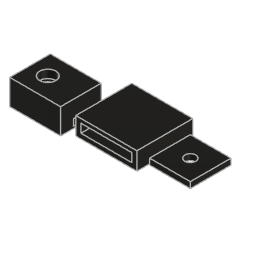
fit-coupons (Autodesk Fusion 360 design; units mm, degrees)
description: Fit sample only; a 25 mm screw will protrude through this shorter coupon
description: Insert measured acrylic from the open end; check emitting centre against edge
description: Test the actual printed reset stem in this 4.3 mm bore
Autodesk Fusion 360 part; units mm, degrees
sketch "Fastener test block profile" plane through (0, 0, 0) normal (0, 0, 1) x (1, 0, 0) in component "90 M3 head and nut fit sample"
  line L0 (0, 0) -> (20, 0)
  line L1 (20, 0) -> (20, 16)
  line L2 (20, 16) -> (0, 16)
  line L3 (0, 16) -> (0, 0)
  dimension "d44" = 20
  dimension "d45" = 16
  measures "d44" horizontal distance of L0.start L0.end
  measures "d45" vertical distance of L0.end L1.end
extrude "Fastener test block" add sketch "Fastener test block profile" against normal blind 10 makes body 1 in component "90 M3 head and nut fit sample"
sketch "M3 clearance profile" plane through (0, 0, 0) normal (0, 0, 1) x (1, 0, 0) in component "90 M3 head and nut fit sample"
  circle A0 centre (7, 8) radius 1.7
  dimension "d48" = 3.4
  measures "d48" diameter of A0
extrude "M3 clearance" cut sketch "M3 clearance profile" against normal blind 10 bodies 1 in component "90 M3 head and nut fit sample"
sketch "M3 head recess profile" plane through (0, 0, 0) normal (0, 0, 1) x (1, 0, 0) in component "90 M3 head and nut fit sample"
  circle A0 centre (7, 8) radius 3.2
  dimension "d51" = 6.4
  measures "d51" diameter of A0
extrude "M3 head recess" cut sketch "M3 head recess profile" against normal blind 3.2 bodies 1 in component "90 M3 head and nut fit sample"
ref_plane "WorkPlane1" through (0, 0, -6.6) normal (0, 0, 1) x (1, 0, 0) in component "90 M3 head and nut fit sample"
sketch "Nut sample hex" plane through (0, 0, -6.6) normal (0, 0, 1) x (1, 0, 0) in component "90 M3 head and nut fit sample"
  line L0 (10.3486, 8) -> (8.6743, 10.9)
  line L1 (8.6743, 10.9) -> (5.3257, 10.9)
  line L2 (5.3257, 10.9) -> (3.6514, 8)
  line L3 (3.6514, 8) -> (5.3257, 5.1)
  line L4 (5.3257, 5.1) -> (8.6743, 5.1)
  line L5 (8.6743, 5.1) -> (10.3486, 8)
extrude "Nut pocket" cut sketch "Nut sample hex" against normal blind 2.6 bodies 1 in component "90 M3 head and nut fit sample"
ref_plane "WorkPlane2" through (0, 0, -6.6) normal (0, 0, 1) x (1, 0, 0) in component "90 M3 head and nut fit sample"
sketch "Side nut loading slot profile" plane through (0, 0, -6.6) normal (0, 0, 1) x (1, 0, 0) in component "90 M3 head and nut fit sample"
  line L0 (7, 5.1) -> (20, 5.1)
  line L1 (20, 5.1) -> (20, 10.9)
  line L2 (20, 10.9) -> (7, 10.9)
  line L3 (7, 10.9) -> (7, 5.1)
  dimension "d60" = 13
  dimension "d61" = 5.8
  measures "d60" horizontal distance of L0.start L0.end
  measures "d61" vertical distance of L0.end L1.end
extrude "Side nut loading slot" cut sketch "Side nut loading slot profile" against normal blind 2.6 bodies 1 in component "90 M3 head and nut fit sample"
sketch "Optical test block profile" plane through (0, 0, 0) normal (0, 0, 1) x (1, 0, 0) in component "91 LED and acrylic fit sample"
  line L0 (26, 0) -> (50, 0)
  line L1 (50, 0) -> (50, 22)
  line L2 (50, 22) -> (26, 22)
  line L3 (26, 22) -> (26, 0)
  dimension "d64" = 24
  dimension "d65" = 22
  measures "d64" horizontal distance of L0.start L0.end
  measures "d65" vertical distance of L0.end L1.end
extrude "Optical test block" add sketch "Optical test block profile" against normal blind 7 separate body makes body 2 in component "91 LED and acrylic fit sample"
ref_plane "WorkPlane1" through (0, 0, -1.6) normal (0, 0, 1) x (1, 0, 0) in component "91 LED and acrylic fit sample"
sketch "Acrylic slip slot profile" plane through (0, 0, -1.6) normal (0, 0, 1) x (1, 0, 0) in component "91 LED and acrylic fit sample"
  line L0 (28, -0.1) -> (48, -0.1)
  line L1 (48, -0.1) -> (48, 12.2)
  line L2 (48, 12.2) -> (28, 12.2)
  line L3 (28, 12.2) -> (28, -0.1)
  dimension "d70" = 20
  dimension "d71" = 12.3
  measures "d70" horizontal distance of L0.start L0.end
  measures "d71" vertical distance of L0.end L1.end
extrude "Acrylic slip slot" cut sketch "Acrylic slip slot profile" against normal blind 3.425 bodies 2 in component "91 LED and acrylic fit sample"
ref_plane "WorkPlane2" through (0, 0, -2.1875) normal (0, 0, 1) x (1, 0, 0) in component "91 LED and acrylic fit sample"
sketch "LED open rear pocket profile" plane through (0, 0, -2.1875) normal (0, 0, 1) x (1, 0, 0) in component "91 LED and acrylic fit sample"
  line L0 (33.8, 12.2) -> (42.2, 12.2)
  line L1 (42.2, 12.2) -> (42.2, 20.6)
  line L2 (42.2, 20.6) -> (33.8, 20.6)
  line L3 (33.8, 20.6) -> (33.8, 12.2)
  dimension "d76" = 8.4
  dimension "d77" = 8.4
  measures "d76" horizontal distance of L0.start L0.end
  measures "d77" vertical distance of L0.end L1.end
extrude "LED open rear pocket" cut sketch "LED open rear pocket profile" against normal blind 5 bodies 2 in component "91 LED and acrylic fit sample"
ref_plane "WorkPlane3" through (0, 0, -1.6) normal (0, 0, 1) x (1, 0, 0) in component "91 LED and acrylic fit sample"
sketch "Optical entry aperture profile" plane through (0, 0, -1.6) normal (0, 0, 1) x (1, 0, 0) in component "91 LED and acrylic fit sample"
  line L0 (33.8, 11.9) -> (42.2, 11.9)
  line L1 (42.2, 11.9) -> (42.2, 12.3)
  line L2 (42.2, 12.3) -> (33.8, 12.3)
  line L3 (33.8, 12.3) -> (33.8, 11.9)
  dimension "d82" = 8.4
  dimension "d83" = 0.4
  measures "d82" horizontal distance of L0.start L0.end
  measures "d83" vertical distance of L0.end L1.end
extrude "Optical entry aperture" cut sketch "Optical entry aperture profile" against normal blind 3.425 bodies 2 in component "91 LED and acrylic fit sample"
sketch "Plunger guide block profile" plane through (0, 0, 0) normal (0, 0, 1) x (1, 0, 0) in component "92 Reset guide fit sample"
  line L0 (55, 0) -> (71, 0)
  line L1 (71, 0) -> (71, 16)
  line L2 (71, 16) -> (55, 16)
  line L3 (55, 16) -> (55, 0)
  dimension "d86" = 16
  dimension "d87" = 16
  measures "d86" horizontal distance of L0.start L0.end
  measures "d87" vertical distance of L0.end L1.end
extrude "Plunger guide block" add sketch "Plunger guide block profile" against normal blind 2.4 separate body makes body 3 in component "92 Reset guide fit sample"
sketch "Stem guide clearance profile" plane through (0, 0, 0) normal (0, 0, 1) x (1, 0, 0) in component "92 Reset guide fit sample"
  circle A0 centre (63, 8) radius 2.15
  dimension "d90" = 4.3
  measures "d90" diameter of A0
extrude "Stem guide clearance" cut sketch "Stem guide clearance profile" against normal blind 2.4 bodies 3 in component "92 Reset guide fit sample"
component "90 M3 head and nut fit sample" placed x (1, 0, 0) y (0, 1, 0) z (0, 0, 1) at (0, 0, 0)
component "91 LED and acrylic fit sample" placed x (1, 0, 0) y (0, 1, 0) z (0, 0, 1) at (0, 0, 0)
component "92 Reset guide fit sample" placed x (1, 0, 0) y (0, 1, 0) z (0, 0, 1) at (0, 0, 0)
equation "case_w = 120.0000000 mm" comment "Overall width"
equation "case_h = 60.0000000 mm" comment "Overall height"
equation "case_d = 30.0000000 mm" comment "Overall depth; excludes adhesive strips"
equation "wall = 2.4000000 mm" comment "PETG wall thickness"
equation "front_lip = 1.6000000 mm" comment "Front retaining lip"
equation "window_w = 100.0000000 mm" comment "Visible opening width"
equation "window_h = 34.0000000 mm" comment "Visible opening height"
equation "panel_w = 104.0000000 mm" comment "Keyed optical panel width"
equation "panel_h = 38.0000000 mm" comment "Keyed optical panel height"
equation "acrylic_t = 3.1750000 mm" comment "MEASURE: actual sheet thickness"
equation "air_gap = 0.5000000 mm" comment "Clearance from engraving to raised white letters"
equation "backing_base = 1.6000000 mm" comment "Black backing base thickness"
equation "letter_relief = 0.4000000 mm" comment "White final two 0.2 mm layers"
equation "tray_t = 1.6000000 mm" comment "Optical support and electronics tray base"
equation "fit = 0.2500000 mm" comment "Sliding fit allowance per side; verify with coupon"
equation "led_w = 8.0000000 mm" comment "MEASURE: individual LED PCB width"
equation "led_h = 8.0000000 mm" comment "MEASURE: individual LED PCB length"
equation "led_t = 2.0000000 mm" comment "MEASURE: LED assembly depth"
equation "led_face_gap = 0.2000000 mm" comment "Emitter to acrylic edge gap"
equation "led_optical_offset = 1.0000000 mm" comment "MEASURE: emitter centre from frontmost module surface"
equation "battery_w = 52.0000000 mm" comment "Supplied battery width"
equation "battery_h = 21.0000000 mm" comment "Supplied battery height"
equation "battery_t = 10.0000000 mm" comment "Supplied battery thickness"
equation "charger_w = 16.5000000 mm" comment "Listed board width; confirm physical board"
equation "charger_h = 25.0000000 mm" comment "Listed board length; confirm physical board"
equation "charger_pcb_t = 1.0000000 mm" comment "MEASURE: charging PCB thickness"
equation "charger_component_t = 4.5000000 mm" comment "RESERVED: component-side envelope"
equation "xiao_length = 21.0000000 mm" comment "Seeed PCB length along case height"
equation "xiao_width = 17.8000000 mm" comment "Seeed PCB width along case depth"
equation "xiao_pcb_t = 1.0000000 mm" comment "MEASURE: XIAO PCB thickness"
equation "reset_y = 54.7000000 mm" comment "MEASURE: reset centre height in installed orientation"
equation "reset_depth = 12.3000000 mm" comment "MEASURE: reset centre depth in installed orientation"
equation "reset_tip_x = 114.1000000 mm" comment "MEASURE: resting contact tip; tune using coupon"
equation "reset_stroke = 0.5000000 mm" comment "PROVISIONAL: total plunger travel including free play"
equation "switch_w = 8.6000000 mm" comment "DPDT body length"
equation "switch_h = 3.1000000 mm" comment "DPDT body width"
equation "switch_t = 2.7000000 mm" comment "DPDT body depth"
equation "switch_throw = 2.0000000 mm" comment "MEASURE: lateral DPDT throw; 1.4 mm is actuator height"
equation "m3_hole = 3.4000000 mm" comment "M3 clearance diameter"
equation "head_d = 6.4000000 mm" comment "Socket head pocket diameter"
equation "head_depth = 3.2000000 mm" comment "Screw head pocket depth"
equation "nut_af = 5.8000000 mm" comment "M3 hex pocket across flats"
equation "text_h = 18.0000000 mm" comment "Native Fusion text height; same master for both optical layers"
equation "d48 = m3_hole"
equation "d51 = head_d"
named bodies: "Fastener test block", "Optical test block", "Plunger guide block"
